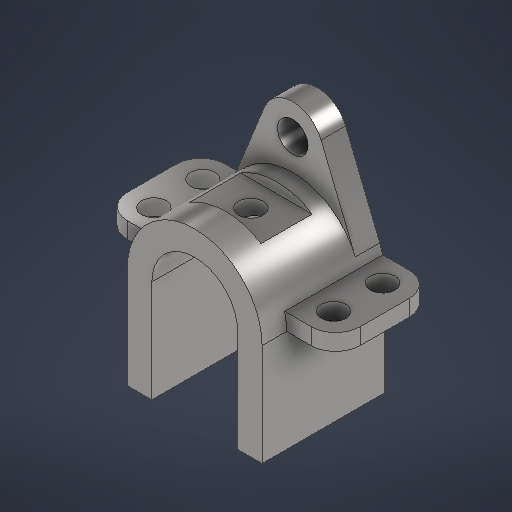
# Autodesk Inventor part: Pieza15
Saved by Autodesk Inventor 2026.2 (Build 302298000, 298)
## iProperties
Created: 2025-12-24
Part Number: Pieza15
Material: Acero inoxidable
Document SubType Name: Modeling
Designer: vicho
Mass: 1236.66 g
Surface Area: 366.481 cm^2
Volume: 154.582 cm^3
Density: 8 g/cm^3
Appearance: Semipulido
Author: vicho
Autodesk Inventor part; units mm, degrees
ref_plane "YZ Plane" through (0, 0, 0) normal (1, 0, 0) x (0, 1, 0)
ref_plane "XY Plane" through (0, 0, 0) normal (0, 0, 1) x (1, 0, 0)
sketch "Boceto1" plane through (0, 0, 0) normal (0, 0, 1) x (1, 0, 0)
  line L0 (0, 100) -> (0, -100) construction
  line L1 (-100, 0) -> (100, 0) construction
  line L2 (-21, -50) -> (-21, 0)
  line L3 (21, -50) -> (21, 0)
  arc A0 (21, 0) -> (-21, 0) centre (0, 0) ccw
  arc A1 (33, 0) -> (-33, 0) centre (0, 0) ccw
  line L4 (-33, 0) -> (-33, -50)
  line L5 (33, 0) -> (33, -50)
  line L6 (-21, -50) -> (-33, -50)
  line L7 (21, -50) -> (33, -50)
  circle A2 centre (0, 48) radius 7.5
  arc A3 (13.9054, 53.625) -> (-13.9054, 53.625) centre (0, 48) ccw
  line L8 (-13.9054, 53.625) -> (-30.5918, 12.375)
  line L9 (13.9054, 53.625) -> (30.5918, 12.375)
  line L10 (-33, 0) -> (-57, 0)
  line L11 (-57, 0) -> (-57, 8)
  line L12 (-57, 8) -> (-32.0156, 8)
  line L13 (100, 0) -> (-100, 0) construction
  line L14 (33, 0) -> (57, 0)
  line L15 (57, 0) -> (57, 8)
  line L16 (57, 8) -> (32.0156, 8)
  point P0 (0, 33)
  dimension "d0" = 200
  dimension "d1" = 200
  dimension "d2" = 50
  dimension "d3" = 50
  dimension "d4" = 42
  dimension "d5" = 33
  dimension "d6" = 15
  dimension "d7" = 48
  dimension "d8" = 15
  dimension "d9" = 24
  dimension "d10" = 8
  dimension "d26" = 33
  constraints: 34 end point, 10 point on circle, 8 point on line, 7 symmetric about line, 5 vertical, 4 centre point, 4 horizontal, 4 tangent, 3 coincident, 3 perpendicular, 2 midpoint, 1 other
  measures "d0" distance of L0.end L0.start
  measures "d1" distance of L1.end L1.start
  measures "d2" distance of L2.start L2.end
  measures "d3" distance of L3.start L3.end
  measures "d4" distance between parallel lines of L3 L2
  measures "d5" radius of A1
  measures "d6" diameter of A2
  measures "d7" distance of point (0, 0) A2.centre
  measures "d8" radius of A3
  measures "d9" distance from line of L4.start L11
  measures "d10" distance of L10.end L11.end
  measures "d26" distance of point (0, 33) point (0, 0)
extrude "Extrusión1" add sketch "Boceto1" along normal blind 60 contours L6 L4 A1 L5 L7 L3 A0 L2
extrude "Extrusión2" add sketch "Boceto1" along normal blind 12 contours L8 A3 L9 A1
extrude "Extrusión3" add sketch "Boceto1" along normal blind 48 contours L10 L11 L12 A1 | A1 L16 L15 L14
fillet "Empalme1" radius 12 4 edges at (57, 4, 48) (-57, 4, 48) (57, 4, 0) (-57, 4, 0)
sketch "Boceto2" plane through (32.0156, 8, 48) normal (0, 1, 0) x (1, 0, 0)
  line L0 (12.9844, 0) -> (0, 0) projected
  line L1 (12.9844, 48) -> (0, 48) projected
  line L2 (0, 0) -> (0, 48) projected
  circle A0 centre (12, 36) radius 6
  circle A1 centre (12, 12) radius 6
  line L3 (-32.0156, 86.4506) -> (-32.0156, -39.8075) construction
  circle A2 centre (-76.0312, 36) radius 6
  circle A3 centre (-76.0312, 12) radius 6
  point P0 (-32.0156, 48)
  dimension "d18" = 12
  dimension "d19" = 12
  dimension "d20" = 12
  dimension "d21" = 12
  dimension "d22" = 12
  dimension "d23" = 12
  constraints: 4 centre point, 2 coincident, 2 end point, 2 symmetric about line, 2 vertical, 2 other
  measures "d18" distance from line of L0 point (12, 12)
  measures "d19" distance from line of L1 point (12, 36)
  measures "d20" distance from line of L2 point (12, 36)
  measures "d21" distance from line of L2 point (12, 12)
  measures "d22" diameter of A0
  measures "d23" diameter of A1
extrude "Extrusión4" cut sketch "Boceto2" against normal blind 48
ref_plane "Plano de trabajo1" through (0, 33, 0) normal (0, 1, 0) x (-1, 0, 0)
sketch "Boceto3" plane through (0, 33, 0) normal (0, 1, 0) x (-1, 0, 0)
  line L0 (-17.465, 45) -> (17.465, 45)
  line L1 (17.465, 45) -> (17.465, 20)
  line L2 (17.465, 20) -> (-17.465, 20)
  line L3 (-17.465, 20) -> (-17.465, 45)
  line L4 (-17.465, 45) -> (17.465, 20) construction
  line L5 (17.465, 45) -> (-17.465, 20) construction
  line L6 (13.9054, 12) -> (-13.9054, 12) projected
  line L7 (0, -11.8316) -> (0, 73.0134) construction
  circle A0 centre (0, 32.5) radius 6
  point P0 (0, 0)
  dimension "d28" = 8
  dimension "d29" = 25
  dimension "d30" = 34.93
  dimension "d31" = 12
  constraints: 14 end point, 2 midpoint, 2 parallel, 2 vertical, 1 centre point, 1 coincident, 1 horizontal, 1 perpendicular, 1 other
  measures "d28" distance between parallel lines of L2 L6
  measures "d29" distance of L0.end L1.end
  measures "d30" distance of L0.start L0.end
  measures "d31" diameter of A0
extrude "Extrusión5" cut sketch "Boceto3" against normal blind 5
extrude "Extrusión6" cut sketch "Boceto3" against normal blind 20 contours A0
